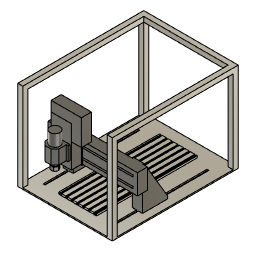
FluidNC Refit Machine Model (Autodesk Fusion 360 design; units mm, degrees)
Autodesk Fusion 360 part; units mm, degrees
sketch "Sketch1" plane through (0, 0, 0) normal (0, 0, 1) x (1, 0, 0) in component "base"
  line L0 (-100, -100) -> (650, -100)
  line L1 (650, -100) -> (650, 900)
  line L2 (650, 900) -> (-100, 900)
  line L3 (-100, 900) -> (-100, -100)
  dimension "d1" = 750
  dimension "d2" = 1000
  dimension "d3" = 100
  dimension "d4" = 100
  constraint horizontal L0
  constraint vertical L1
  constraint horizontal L2
  constraint vertical L3
  measures "d1" distance of L0.start L0.end
  measures "d2" distance of L0.start L2.end
  measures "d3" distance of origin L3
  measures "d4" distance of origin L0
extrude "Extrude1" add sketch "Sketch1" against normal blind 10 makes body 1 in component "base"
ref_plane "WorkPlane1" through (275, 400, -5) normal (-1, 0, 0) x (0, 1, 0)
ref_plane "WorkPlane2" through (275, 400, -5) normal (0, 1, 0) x (1, 0, 0)
sketch "Sketch2" plane through (0, 0, 0) normal (0, 1, 0) x (1, 0, 0) in component "base"
  line L0 (0, 0) -> (125, 0) construction
  line L1 (125, 0) -> (425, 0)
  line L2 (650, 10) -> (-100, 10) construction
  line L3 (275, 0) -> (275, 10) construction
  line L4 (425, 0) -> (425, -15)
  line L5 (425, -15) -> (125, -15) construction
  line L6 (125, -15) -> (125, 0)
  line L7 (275, 0) -> (275, -15) construction
  line L8 (279.15, -15) -> (279.15, -10.6)
  line L9 (279.15, -10.6) -> (282.5, -10.6)
  line L10 (282.5, -10.6) -> (282.5, -4.4)
  line L11 (282.5, -4.4) -> (267.5, -4.4)
  line L12 (267.5, -4.4) -> (267.5, -10.6)
  line L13 (267.5, -10.6) -> (270.85, -10.6)
  line L14 (270.85, -10.6) -> (270.85, -15)
  line L15 (270.85, -10.6) -> (279.15, -10.6) construction
  line L16 (279.15, -15) -> (297.5, -15)
  line L17 (270.85, -15) -> (252.5, -15)
  line L18 (144.15, -15) -> (162.5, -15)
  line L19 (144.15, -15) -> (144.15, -10.6)
  line L20 (144.15, -10.6) -> (147.5, -10.6)
  line L21 (147.5, -4.4) -> (132.5, -4.4)
  line L22 (132.5, -4.4) -> (132.5, -10.6)
  line L23 (132.5, -10.6) -> (135.85, -10.6)
  line L24 (135.85, -10.6) -> (135.85, -15)
  line L25 (135.85, -15) -> (117.5, -15)
  line L26 (147.5, -10.6) -> (147.5, -4.4)
  line L27 (189.15, -15) -> (207.5, -15)
  line L28 (189.15, -15) -> (189.15, -10.6)
  line L29 (189.15, -10.6) -> (192.5, -10.6)
  line L30 (192.5, -4.4) -> (177.5, -4.4)
  line L31 (177.5, -4.4) -> (177.5, -10.6)
  line L32 (177.5, -10.6) -> (180.85, -10.6)
  line L33 (180.85, -10.6) -> (180.85, -15)
  line L34 (180.85, -15) -> (162.5, -15)
  line L35 (192.5, -10.6) -> (192.5, -4.4)
  line L36 (234.15, -15) -> (252.5, -15)
  line L37 (234.15, -15) -> (234.15, -10.6)
  line L38 (234.15, -10.6) -> (237.5, -10.6)
  line L39 (237.5, -4.4) -> (222.5, -4.4)
  line L40 (222.5, -4.4) -> (222.5, -10.6)
  line L41 (222.5, -10.6) -> (225.85, -10.6)
  line L42 (225.85, -10.6) -> (225.85, -15)
  line L43 (225.85, -15) -> (207.5, -15)
  line L44 (237.5, -10.6) -> (237.5, -4.4)
  line L45 (324.15, -15) -> (342.5, -15)
  line L46 (324.15, -15) -> (324.15, -10.6)
  line L47 (324.15, -10.6) -> (327.5, -10.6)
  line L48 (327.5, -4.4) -> (312.5, -4.4)
  line L49 (312.5, -4.4) -> (312.5, -10.6)
  line L50 (312.5, -10.6) -> (315.85, -10.6)
  line L51 (315.85, -10.6) -> (315.85, -15)
  line L52 (315.85, -15) -> (297.5, -15)
  line L53 (327.5, -10.6) -> (327.5, -4.4)
  line L54 (369.15, -15) -> (387.5, -15)
  line L55 (369.15, -15) -> (369.15, -10.6)
  line L56 (369.15, -10.6) -> (372.5, -10.6)
  line L57 (372.5, -4.4) -> (357.5, -4.4)
  line L58 (357.5, -4.4) -> (357.5, -10.6)
  line L59 (357.5, -10.6) -> (360.85, -10.6)
  line L60 (360.85, -10.6) -> (360.85, -15)
  line L61 (360.85, -15) -> (342.5, -15)
  line L62 (372.5, -10.6) -> (372.5, -4.4)
  line L63 (414.15, -15) -> (432.5, -15)
  line L64 (414.15, -15) -> (414.15, -10.6)
  line L65 (414.15, -10.6) -> (417.5, -10.6)
  line L66 (417.5, -4.4) -> (402.5, -4.4)
  line L67 (402.5, -4.4) -> (402.5, -10.6)
  line L68 (402.5, -10.6) -> (405.85, -10.6)
  line L69 (405.85, -10.6) -> (405.85, -15)
  line L70 (405.85, -15) -> (387.5, -15)
  line L71 (417.5, -10.6) -> (417.5, -4.4)
  point P0 (275, -4.4)
  point P1 (275, -10.6)
  dimension "d7" = 300
  dimension "d8" = 15
  dimension "d9" = 8.3
  dimension "d10" = 10.6
  dimension "d11" = 4.4
  dimension "d12" = 15
  dimension "d13" = 45
  dimension "d16" = 45
  dimension "d17" = 0
  constraint coincident L0.start origin
  constraint horizontal L0
  constraint parallel L0 L1
  constraint midpoint L1 L3.start
  constraint midpoint L2 L3.end
  constraint perpendicular L1 L3
  constraint perpendicular L1 L4
  constraint perpendicular L4 L5
  constraint perpendicular L1 L6
  constraint midpoint L5 L7.end
  constraint coincident L5 L8.start
  constraint perpendicular L5 L8
  constraint perpendicular L8 L9
  constraint perpendicular L5 L10
  constraint perpendicular L7 L11
  constraint perpendicular L11 L12
  constraint perpendicular L12 L13
  constraint coincident L5 L14.end
  constraint perpendicular L5 L14
  constraint perpendicular L8 L15
  constraint midpoint L11 P0
  constraint midpoint L15 P1
  constraint coincident L7 P1
  constraint coincident L7 P0
  constraint coincident L5 L16.end
  constraint coincident L5 L17.end
  constraint equal L16 L17
  measures "d7" distance of L0.end L1.end
  measures "d8" distance of L1.end L4.end
  measures "d9" distance of L8 L14
  measures "d10" distance of L5 L11
  measures "d11" distance of L5 L13
  measures "d12" distance of L10 L12
  measures "d13" distance of L16.end L17.end
extrude "Extrude2" add sketch "Sketch2" along normal blind 800 bodies 1 in component "base"
sketch "Sketch3" plane through (0, 0, 0) normal (0, 0, 1) x (-1, 0, 0) in component "base"
  line L0 (-425, -800) -> (-425, 0)
  line L1 (-425, 0) -> (-125, 0)
  line L2 (-125, 0) -> (-125, -800)
  line L3 (-125, -800) -> (-425, -800)
  line L4 (100, -900) -> (100, 100)
  line L5 (100, 100) -> (-650, 100)
  line L6 (-650, 100) -> (-650, -900)
  line L7 (-650, -900) -> (100, -900)
  line L8 (100, -900) -> (60, -900)
  line L9 (60, -900) -> (60, -860)
  line L10 (60, -860) -> (100, -860)
  line L11 (100, -860) -> (100, -900)
  line L12 (-650, -900) -> (-610, -900)
  line L13 (-610, -900) -> (-610, -860)
  line L14 (-610, -860) -> (-650, -860)
  line L15 (-650, -860) -> (-650, -900)
  line L16 (-650, 100) -> (-610, 100)
  line L17 (-610, 100) -> (-610, 60)
  line L18 (-610, 60) -> (-650, 60)
  line L19 (-650, 60) -> (-650, 100)
  line L20 (100, 100) -> (60, 100)
  line L21 (60, 100) -> (60, 60)
  line L22 (60, 60) -> (100, 60)
  line L23 (100, 60) -> (100, 100)
  line L24 (60, -860) -> (-610, -860) construction
  line L25 (-610, -860) -> (-610, 60) construction
  line L26 (-610, 60) -> (60, 60) construction
  line L27 (60, 60) -> (60, -860) construction
  dimension "d21" = 40
  constraint horizontal L8
  constraint vertical L9
  constraint horizontal L10
  constraint vertical L11
  constraint coincident L4.start L7.end
  constraint horizontal L12
  constraint vertical L13
  constraint horizontal L14
  constraint vertical L15
  constraint coincident L6.end L7.start
  constraint horizontal L16
  constraint vertical L17
  constraint horizontal L18
  constraint vertical L19
  constraint coincident L5.end L6.start
  constraint horizontal L20
  constraint vertical L21
  constraint horizontal L22
  constraint vertical L23
  constraint coincident L4.end L5.start
  constraint horizontal L24
  constraint vertical L25
  constraint horizontal L26
  constraint vertical L27
  constraint coincident L13.end L14.start
  constraint equal L8 L11
  constraint equal L12 L15
  constraint equal L20 L23
  constraint coincident L21.end L22.start
  measures "d21" distance of L4.start L10.end
extrude "Extrude3" add sketch "Sketch3" along normal blind 700 contours L4 L7 L8 L9 L10 L11 | L4 L5 L20 L21 L22 L23 | L6 L7 L12 L13 L14 L15 | L5 L6 L16 L17 L18 L19 bodies 1 in component "base"
sketch "Sketch4" plane through (0, 860, 0) normal (0, -1, 0) x (1, 0, 0) in component "base"
  line L0 (-100, 0) -> (-60, 0)
  line L1 (-60, 0) -> (-60, 700)
  line L2 (-60, 700) -> (-100, 700)
  line L3 (-100, 700) -> (-100, 0)
  line L4 (-100, 700) -> (-60, 700)
  line L5 (-60, 700) -> (-60, 660)
  line L6 (-60, 660) -> (-100, 660)
  line L7 (-100, 660) -> (-100, 700)
  line L8 (610, 700) -> (650, 700) construction
  line L9 (610, 700) -> (650, 700)
  line L10 (650, 700) -> (650, 660)
  line L11 (650, 660) -> (610, 660)
  line L12 (610, 660) -> (610, 700)
  constraint horizontal L4
  constraint vertical L5
  constraint horizontal L6
  constraint vertical L7
  constraint coincident L1 L5.end
  constraint coincident L2.end L3.start
  constraint equal L4 L7
  constraint horizontal L9
  constraint vertical L10
  constraint horizontal L11
  constraint vertical L12
  constraint coincident L8.start L9.start
  constraint coincident L5.end L11
  constraint coincident L8.end L10
extrude "Extrude4" add sketch "Sketch4" along normal blind 920 contours L1 L2 L3 L4 L5 L6 L7 | L9 L10 L11 L12 bodies 1 in component "base"
sketch "Sketch5" plane through (610, 0, 0) normal (-1, 0, 0) x (0, -1, 0) in component "base"
  line L0 (-900, 0) -> (-860, 0)
  line L1 (-860, 0) -> (-860, 660)
  line L2 (-860, 660) -> (60, 660)
  line L3 (60, 660) -> (60, 0)
  line L4 (60, 0) -> (100, 0)
  line L5 (100, 0) -> (100, 700)
  line L6 (100, 700) -> (-900, 700)
  line L7 (-900, 700) -> (-900, 0)
  line L8 (-860, 660) -> (-900, 660)
  line L9 (-860, 660) -> (-860, 700)
  line L10 (60, 660) -> (60, 700)
  line L11 (60, 660) -> (100, 660)
  constraint coincident L1.end L2.start
  constraint coincident L7 L8.end
  constraint perpendicular L7 L8
  constraint coincident L6 L9.end
  constraint perpendicular L6 L9
  constraint coincident L2.end L3.start
  constraint coincident L6 L10.end
  constraint perpendicular L6 L10
  constraint coincident L5 L11.end
  constraint perpendicular L5 L11
extrude "Extrude5" add sketch "Sketch5" along normal blind 670 contours L6 L7 L8 L9 bodies 1 in component "base"
sketch "Sketch6" plane through (0, 0, 0) normal (0, 0, 1) x (-1, 0, 0) in component "base"
  line L0 (-610, -860) -> (-610, -900)
  line L1 (-610, -900) -> (60, -900)
  line L2 (60, -900) -> (60, -860)
  line L3 (60, -860) -> (100, -860)
  line L4 (100, -860) -> (100, 60)
  line L5 (100, 60) -> (60, 60)
  line L6 (60, 60) -> (60, 100)
  line L7 (60, 100) -> (-610, 100)
  line L8 (-610, 60) -> (-650, 60)
  line L9 (-650, 60) -> (-650, -860)
  line L10 (-650, -860) -> (-610, -860)
  line L11 (-425, -800) -> (-425, 0)
  line L12 (-425, 0) -> (-125, 0)
  line L13 (-125, 0) -> (-125, -800)
  line L14 (-125, -800) -> (-425, -800)
  line L15 (7.5, -10) -> (-7.5, -10)
  line L16 (-7.5, -10) -> (-7.5, -760)
  line L17 (-7.5, -760) -> (7.5, -760)
  line L18 (7.5, -760) -> (7.5, -10)
  line L19 (-275, 100) -> (-275, -900) construction
  line L20 (-542.5, -10) -> (-542.5, -760)
  line L21 (-542.5, -760) -> (-557.5, -760)
  line L22 (-557.5, -10) -> (-542.5, -10)
  line L23 (-557.5, -760) -> (-557.5, -10)
  line L24 (-610, 100) -> (-610, 60)
  dimension "d28" = 15
  dimension "d29" = 750
  dimension "d30" = 92.5
  dimension "d31" = 110
  constraint horizontal L15
  constraint vertical L16
  constraint horizontal L17
  constraint vertical L18
  constraint midpoint L7 L19.start
  constraint midpoint L1 L19.end
  constraint symmetric L15.start L19 L22.start
  constraint symmetric L15.end L19 L20.start
  constraint symmetric L16.end L19 L20.end
  constraint symmetric L17.end L19 L21.end
  measures "d28" distance of L15.start L15.end
  measures "d29" distance of L15.start L17.end
  measures "d30" distance of L4 L18
  measures "d31" distance of L7 L15
extrude "Extrude6" cut sketch "Sketch6" against normal blind 10 contours L15 L16 L17 L18 | L20 L21 L22 L23 bodies 1 in component "base"
sketch "Sketch7" plane through (0, 0, 0) normal (0, 0, 1) x (-1, 0, 0) in component "base"
  line L0 (-7.5, -10) -> (7.5, -10)
  line L1 (7.5, -10) -> (7.5, -760)
  line L2 (7.5, -760) -> (-7.5, -760)
  line L3 (-7.5, -760) -> (-7.5, -10)
  line L4 (-542.5, -10) -> (-542.5, -760)
  line L5 (-542.5, -760) -> (-557.5, -760)
  line L6 (-557.5, -760) -> (-557.5, -10)
  line L7 (-557.5, -10) -> (-542.5, -10)
  line L8 (-610, -860) -> (-610, -900)
  line L9 (-610, -900) -> (60, -900)
  line L10 (60, -900) -> (60, -860)
  line L11 (60, -860) -> (100, -860)
  line L12 (100, -860) -> (100, 60)
  line L13 (100, 60) -> (60, 60)
  line L14 (60, 60) -> (60, 100)
  line L15 (60, 100) -> (-610, 100)
  line L16 (-610, 60) -> (-650, 60)
  line L17 (-650, 60) -> (-650, -860)
  line L18 (-650, -860) -> (-610, -860)
  line L19 (-425, -800) -> (-425, 0)
  line L20 (-425, 0) -> (-125, 0)
  line L21 (-125, 0) -> (-125, -800)
  line L22 (-125, -800) -> (-425, -800)
  line L23 (80, -860) -> (80, 60) construction
  line L24 (-630, 60) -> (-630, -860) construction
  line L25 (-610, -880) -> (60, -880) construction
  line L26 (-610, -885) -> (60, -885)
  line L27 (60, -885) -> (60, -875)
  line L28 (60, -875) -> (-610, -875)
  line L29 (-610, -875) -> (-610, -885)
  line L30 (-610, -885) -> (60, -875) construction
  line L31 (60, -885) -> (-610, -875) construction
  line L32 (-635, -860) -> (-625, -860)
  line L33 (-625, -860) -> (-625, 60)
  line L34 (-625, 60) -> (-635, 60)
  line L35 (-635, 60) -> (-635, -860)
  line L36 (-635, -860) -> (-625, 60) construction
  line L37 (-625, -860) -> (-635, 60) construction
  line L38 (85, -860) -> (75, -860)
  line L39 (75, -860) -> (75, 60)
  line L40 (75, 60) -> (85, 60)
  line L41 (85, 60) -> (85, -860)
  line L42 (85, -860) -> (75, 60) construction
  line L43 (75, -860) -> (85, 60) construction
  line L44 (-610, 100) -> (-610, 60)
  point P0 (-275, -880)
  point P1 (-630, -400)
  point P2 (80, -400)
  dimension "d34" = 10
  dimension "d35" = 670
  dimension "d36" = 10
  dimension "d37" = 10
  constraint midpoint L11 L23.start
  constraint midpoint L13 L23.end
  constraint midpoint L16 L24.start
  constraint midpoint L18 L24.end
  constraint midpoint L8 L25.start
  constraint midpoint L10 L25.end
  constraint horizontal L26
  constraint perpendicular L26 L27
  constraint parallel L26 L28
  constraint parallel L27 L29
  constraint coincident L30 P0
  constraint coincident L31 P0
  constraint midpoint L25 P0
  constraint horizontal L32
  constraint perpendicular L32 L33
  constraint parallel L32 L34
  constraint parallel L33 L35
  constraint coincident L36 P1
  constraint coincident L37 P1
  constraint coincident L18 L32.start
  constraint midpoint L24 P1
  constraint horizontal L38
  constraint perpendicular L38 L39
  constraint parallel L38 L40
  constraint parallel L39 L41
  constraint coincident L42 P2
  constraint coincident L43 P2
  constraint coincident L11 L38.start
  constraint midpoint L23 P2
  measures "d34" distance of L26.end L27.end L40.end
  measures "d35" distance of L26.start L26.end
  measures "d36" distance of L32.start L32.end
  measures "d37" distance of L38.start L38.end
extrude "Extrude7" add sketch "Sketch7" along normal blind 660 separate body contours L8 L10 L26 L27 L28 L29 | L16 L18 L32 L33 L34 L35 | L11 L13 L38 L39 L40 L41 makes body 2 at (-85, 246.6667, 220) makes body 3 at (163.3333, 875, 220) makes body 4 at (635, 246.6667, 220) in component "base"
sketch "Sketch1 (2)" plane through (0, 0, 0) normal (1, 0, 0) x (0, 1, 0) in component "y_axis_head"
  line L0 (200, 0) -> (200, 340)
  line L1 (200, 340) -> (210, 340)
  line L2 (210, 340) -> (400, 20)
  line L3 (400, 20) -> (400, 0)
  line L4 (400, 0) -> (200, 0)
  dimension "d40" = 20
  dimension "d41" = 10
  dimension "d42" = 200
  dimension "d43" = 340
  dimension "d50" = 200
  constraint vertical L0
  constraint perpendicular L0 L1
  constraint vertical L3
  constraint perpendicular L0 L4
  constraint coincident L0.start L4.end
  constraint coincident origin L4
  measures "d40" distance of L2.end L3.end
  measures "d41" distance of L0.end L1.end
  measures "d42" distance of L3.end L0.start
  measures "d43" distance of L0.start L0.end
  measures "d50" distance of origin L0
extrude "Extrude1'" add sketch "Sketch1 (2)" along normal blind 40 and the other way blind 40 separate body makes body 5 in component "y_axis_head"
mirror "Mirror1" about plane through (275, 400, -5) normal (-1, 0, 0) of bodies 5 makes body 6 in component "y_axis_head"
sketch "Sketch3 (2)" plane through (0, 0, 0) normal (1, 0, 0) x (0, 1, 0) in component "y_axis_head"
  line L0 (200, 340) -> (210, 340)
  line L1 (200, 0) -> (200, 340)
  line L2 (200, 340) -> (120, 340)
  line L3 (120, 340) -> (120, 180)
  line L4 (120, 180) -> (200, 180)
  line L5 (200, 180) -> (200, 340)
  dimension "d51" = 80
  dimension "d52" = 160
  constraint horizontal L2
  constraint vertical L3
  constraint horizontal L4
  constraint vertical L5
  constraint coincident L0.start L1.end
  measures "d51" distance of L0.start L2.end
  measures "d52" distance of L0.start L4.end
extrude "Extrude2'" add sketch "Sketch3 (2)" along normal blind 630 and the other way blind 80 bodies 5 6 in component "y_axis_head"
sketch "Sketch4 (2)" plane through (0, 0, 0) normal (0, 0, -1) x (1, 0, 0) in component "y_axis_head"
  line L0 (-40, -400) -> (40, -400)
  line L1 (40, -400) -> (40, -200)
  line L2 (40, -200) -> (-40, -200)
  line L3 (-40, -200) -> (-40, -400)
  line L4 (0, -200) -> (0, -400) construction
  line L5 (7.5, -200) -> (-7.5, -200)
  line L6 (-7.5, -200) -> (-7.5, -400)
  line L7 (-7.5, -400) -> (7.5, -400)
  line L8 (7.5, -400) -> (7.5, -200)
  line L9 (7.5, -200) -> (-7.5, -400) construction
  line L10 (-7.5, -200) -> (7.5, -400) construction
  point P0 (0, -300)
  dimension "d57" = 15
  constraint midpoint L2 L4.start
  constraint midpoint L0 L4.end
  constraint horizontal L5
  constraint perpendicular L5 L6
  constraint parallel L5 L7
  constraint parallel L6 L8
  constraint coincident L9 P0
  constraint coincident L10 P0
  constraint midpoint L4 P0
  constraint coincident L0 L7.end
  measures "d57" distance of L6.end L7.end
extrude "Extrude3'" add sketch "Sketch4 (2)" along normal blind 40 contours L0 L2 L5 L6 L7 L8 bodies 5 in component "y_axis_head"
mirror "Mirror2" about plane through (275, 400, -5) normal (-1, 0, 0) of "Extrude3'" in component "y_axis_head"
sketch "Sketch5 (2)" plane through (0, 120, 0) normal (0, -1, 0) x (1, 0, 0) in component "y_axis_head"
  line L0 (-80, 180) -> (630, 180)
  line L1 (630, 180) -> (630, 340)
  line L2 (630, 340) -> (-80, 340)
  line L3 (-80, 340) -> (-80, 180)
  line L4 (-80, 340) -> (-80, 260) construction
  line L5 (-80, 260) -> (-80, 180) construction
  line L6 (-80, 220) -> (630, 220) construction
  line L7 (-80, 300) -> (630, 300) construction
  line L8 (275, 180) -> (275, 340) construction
  line L9 (595, 292.5) -> (-45, 292.5)
  line L10 (-45, 292.5) -> (-45, 307.5)
  line L11 (-45, 307.5) -> (595, 307.5)
  line L12 (595, 307.5) -> (595, 292.5)
  line L13 (595, 292.5) -> (-45, 307.5) construction
  line L14 (-45, 292.5) -> (595, 307.5) construction
  line L15 (595, 227.5) -> (-45, 227.5)
  line L16 (-45, 227.5) -> (-45, 212.5)
  line L17 (-45, 212.5) -> (595, 212.5)
  line L18 (595, 212.5) -> (595, 227.5)
  line L19 (595, 227.5) -> (-45, 212.5) construction
  line L20 (-45, 227.5) -> (595, 212.5) construction
  point P0 (275, 300)
  point P1 (275, 220)
  dimension "d62" = 640
  dimension "d63" = 15
  constraint coincident L2.end L3.start
  constraint midpoint L3 L4.end
  constraint coincident L0.start L3.end
  constraint midpoint L5 L6.start
  constraint coincident L1 L6.end
  constraint perpendicular L1 L6
  constraint midpoint L4 L7.start
  constraint coincident L1 L7.end
  constraint perpendicular L1 L7
  constraint midpoint L0 L8.start
  constraint midpoint L2 L8.end
  constraint horizontal L9
  constraint perpendicular L9 L10
  constraint parallel L9 L11
  constraint parallel L10 L12
  constraint coincident L13 P0
  constraint coincident L14 P0
  constraint midpoint L7 P0
  constraint horizontal L15
  constraint perpendicular L15 L16
  constraint parallel L15 L17
  constraint parallel L16 L18
  constraint coincident L19 P1
  constraint coincident L20 P1
  constraint midpoint L6 P1
  constraint equal L9 L15
  constraint equal L10 L16
  measures "d62" distance of L10.end L11.end
  measures "d63" distance of L9.end L10.end
extrude "Extrude4'" cut sketch "Sketch5 (2)" against normal blind 20 contours L9 L10 L11 L12 | L15 L16 L17 L18 bodies 5 in component "y_axis_head"
sketch "Sketch1 (3)" plane through (0, 120, 0) normal (0, -1, 0) x (1, 0, 0) in component "x_axis_head"
  line L0 (-45, 292.5) -> (-45, 307.5)
  line L1 (-45, 307.5) -> (595, 307.5)
  line L2 (595, 307.5) -> (595, 292.5)
  line L3 (595, 292.5) -> (-45, 292.5)
  line L4 (-45, 227.5) -> (595, 227.5)
  line L5 (595, 227.5) -> (595, 212.5)
  line L6 (595, 212.5) -> (-45, 212.5)
  line L7 (-45, 212.5) -> (-45, 227.5)
  line L8 (-80, 180) -> (630, 180)
  line L9 (630, 180) -> (630, 340)
  line L10 (630, 340) -> (-80, 340)
  line L11 (-80, 340) -> (-80, 180)
  line L12 (-80, 260) -> (35, 260) construction
  line L13 (35, 260) -> (35, 340) construction
  line L14 (-50, 175) -> (120, 175)
  line L15 (120, 175) -> (120, 345)
  line L16 (120, 345) -> (-50, 345)
  line L17 (-50, 345) -> (-50, 175)
  line L18 (-50, 175) -> (120, 345) construction
  line L19 (120, 175) -> (-50, 345) construction
  line L20 (-45, 300) -> (35, 300) construction
  line L21 (110, 292.5) -> (-40, 292.5)
  line L22 (-40, 292.5) -> (-40, 307.5)
  line L23 (-40, 307.5) -> (110, 307.5)
  line L24 (110, 307.5) -> (110, 292.5)
  line L25 (110, 292.5) -> (-40, 307.5) construction
  line L26 (-40, 292.5) -> (110, 307.5) construction
  line L27 (110, 212.5) -> (110, 227.5)
  line L28 (110, 227.5) -> (-40, 227.5)
  line L29 (-40, 212.5) -> (110, 212.5)
  line L30 (-40, 227.5) -> (-40, 212.5)
  point P0 (35, 260)
  point P1 (35, 300)
  dimension "d66" = 170
  dimension "d67" = 170
  dimension "d70" = 150
  constraint midpoint L11 L12.start
  constraint perpendicular L11 L12
  constraint coincident L10 L13.end
  constraint perpendicular L10 L13
  constraint horizontal L14
  constraint perpendicular L14 L15
  constraint parallel L14 L16
  constraint parallel L15 L17
  constraint coincident L18 P0
  constraint coincident L19 P0
  constraint coincident P0 L12.end
  constraint midpoint L0 L20.start
  constraint perpendicular L13 L20
  constraint equal L13 L20
  constraint coincident L13 P1
  constraint horizontal L21
  constraint perpendicular L21 L22
  constraint parallel L21 L23
  constraint parallel L22 L24
  constraint coincident L25 P1
  constraint coincident L26 P1
  constraint coincident P1 L20.end
  constraint coincident L3 L21.start
  constraint symmetric L12 L21.start L27.end
  constraint symmetric L12 L21.end L28.end
  constraint symmetric L12 L22.end L29.start
  constraint symmetric L12 L23.end L27.start
  measures "d66" distance of L15.end L16.end
  measures "d67" distance of L14.end L15.end
  measures "d70" distance of L22.end L23.end
extrude "Extrude1''" add sketch "Sketch1 (3)" along normal blind 5 separate body contours L0 L1 L3 L4 L6 L7 L8 L10 L15 L17 L21 L23 L28 L29 | L0 L1 L3 L22 | L1 L3 L21 L22 L23 L24 | L1 L3 L15 L24 | L4 L6 L15 L27 | L10 L15 L16 L17 | L4 L6 L27 L28 L29 L30 | L4 L6 L7 L30 | L8 L14 L15 L17 makes body 7 in component "x_axis_head"
extrude "Extrude2''" add sketch "Sketch1 (3)" against normal blind 10 contours L1 L3 L21 L22 L23 L24 | L4 L6 L27 L28 L29 L30 bodies 7 in component "x_axis_head"
sketch "Sketch2 (2)" plane through (0, 115, 0) normal (0, -1, 0) x (1, 0, 0) in component "x_axis_head"
  line L0 (-50, 345) -> (-50, 175)
  line L1 (120, 175) -> (120, 345)
  line L2 (35, 340) -> (35, 180) construction
  line L3 (35, 260) -> (-50, 260) construction
  line L4 (0, 320) -> (-15, 320)
  line L5 (-15, 320) -> (-15, 200)
  line L6 (-15, 200) -> (0, 200)
  line L7 (0, 200) -> (0, 320)
  line L8 (0, 320) -> (-15, 200) construction
  line L9 (-15, 320) -> (0, 200) construction
  line L10 (85, 320) -> (85, 200)
  line L11 (85, 200) -> (70, 200)
  line L12 (70, 320) -> (85, 320)
  line L13 (70, 200) -> (70, 320)
  line L14 (-50, 175) -> (120, 175)
  line L15 (120, 345) -> (-50, 345)
  point P0 (-7.5, 260)
  dimension "d73" = 15
  dimension "d74" = 120
  constraint midpoint L2 L3.start
  constraint midpoint L0 L3.end
  constraint horizontal L4
  constraint perpendicular L4 L5
  constraint parallel L4 L6
  constraint parallel L5 L7
  constraint coincident L8 P0
  constraint coincident L9 P0
  constraint midpoint L3 P0
  constraint symmetric L2 L4.start L12.start
  constraint symmetric L2 L4.end L10.start
  constraint symmetric L2 L5.end L10.end
  constraint symmetric L2 L6.end L11.end
  measures "d73" distance of L5.end L6.end
  measures "d74" distance of L4.end L5.end
extrude "Extrude3''" add sketch "Sketch2 (2)" along normal blind 10 contours L4 L5 L6 L7 | L10 L11 L12 L13 bodies 7 in component "x_axis_head"
sketch "Sketch3 (3)" plane through (0, 115, 0) normal (0, -1, 0) x (1, 0, 0) in component "z_axis_head"
  line L0 (70, 200) -> (70, 320)
  line L1 (70, 320) -> (85, 320)
  line L2 (85, 320) -> (85, 200)
  line L3 (85, 200) -> (70, 200)
  line L4 (0, 200) -> (-15, 200)
  line L5 (-15, 200) -> (-15, 320)
  line L6 (-15, 320) -> (0, 320)
  line L7 (0, 320) -> (0, 200)
  line L8 (-50, 345) -> (-50, 175)
  line L9 (-50, 175) -> (120, 175)
  line L10 (120, 175) -> (120, 345)
  line L11 (120, 345) -> (-50, 345)
  line L12 (-50, 260) -> (120, 260) construction
  line L13 (115, 420) -> (-45, 420)
  line L14 (-45, 420) -> (-45, 100)
  line L15 (-45, 100) -> (115, 100)
  line L16 (115, 100) -> (115, 420)
  line L17 (115, 420) -> (-45, 100) construction
  line L18 (-45, 420) -> (115, 100) construction
  line L19 (-7.5, 320) -> (-7.5, 200) construction
  line L20 (77.5, 320) -> (77.5, 200) construction
  line L21 (0, 400) -> (-15, 400)
  line L22 (-15, 400) -> (-15, 120)
  line L23 (-15, 120) -> (0, 120)
  line L24 (0, 120) -> (0, 400)
  line L25 (0, 400) -> (-15, 120) construction
  line L26 (-15, 400) -> (0, 120) construction
  line L27 (35, 260) -> (35, 420) construction
  line L28 (70, 120) -> (70, 400)
  line L29 (70, 400) -> (85, 400)
  line L30 (85, 120) -> (70, 120)
  line L31 (85, 400) -> (85, 120)
  point P0 (35, 260)
  point P1 (-7.5, 260)
  dimension "d77" = 320
  dimension "d78" = 160
  dimension "d79" = 15
  dimension "d80" = 280
  constraint midpoint L8 L12.start
  constraint midpoint L10 L12.end
  constraint horizontal L13
  constraint perpendicular L13 L14
  constraint parallel L13 L15
  constraint parallel L14 L16
  constraint coincident L17 P0
  constraint coincident L18 P0
  constraint midpoint L12 P0
  constraint midpoint L6 L19.start
  constraint midpoint L4 L19.end
  constraint midpoint L1 L20.start
  constraint midpoint L3 L20.end
  constraint horizontal L21
  constraint perpendicular L21 L22
  constraint parallel L21 L23
  constraint parallel L22 L24
  constraint coincident L25 P1
  constraint coincident L26 P1
  constraint midpoint L19 P1
  constraint coincident P0 L27.start
  constraint midpoint L13 L27.end
  constraint symmetric L21.start L27 L28.end
  constraint symmetric L21.end L27 L29.end
  constraint symmetric L22.end L27 L30.start
  constraint symmetric L23.end L27 L28.start
  measures "d77" distance of L13.end L14.end
  measures "d78" distance of L13.start L13.end
  measures "d79" distance of L22.end L23.end
  measures "d80" distance of L21.end L22.end
extrude "Extrude1'''" add sketch "Sketch3 (3)" along normal blind 80 separate body contours L0 L7 L9 L11 L24 L28 | L0 L1 L2 L3 L28 L31 | L3 L9 L28 L31 | L1 L11 L28 L31 | L2 L9 L11 L16 L31 | L9 L14 L15 L16 L22 L23 L24 L28 L30 L31 | L9 L28 L30 L31 | L11 L28 L29 L31 | L11 L13 L14 L16 L21 L22 L24 L28 L29 L31 | L9 L22 L23 L24 | L4 L9 L22 L24 | L6 L11 L22 L24 | L11 L21 L22 L24 | L5 L9 L11 L14 L22 | L4 L5 L6 L7 L22 L24 makes body 8 in component "z_axis_head"
extrude "Extrude2'''" cut sketch "Sketch3 (3)" along normal blind 10 contours L0 L1 L2 L3 L28 L31 | L3 L9 L28 L31 | L1 L11 L28 L31 | L9 L28 L30 L31 | L11 L28 L29 L31 | L9 L22 L23 L24 | L4 L9 L22 L24 | L6 L11 L22 L24 | L11 L21 L22 L24 | L4 L5 L6 L7 L22 L24 bodies 8 in component "z_axis_head"
sketch "Sketch1 (4)" plane through (0, 0, 100) normal (0, 0, -1) x (1, 0, 0) in component "z_axis_head"
  line L0 (-45, -115) -> (115, -115)
  line L1 (115, -115) -> (115, -35)
  line L2 (115, -35) -> (-45, -35)
  line L3 (-45, -35) -> (-45, -115)
  line L4 (35, -35) -> (35, 15) construction
  circle A0 centre (35, 15) radius 40
  circle A1 centre (35, 15) radius 60 construction
  line L5 (-20, 38.9792) -> (-20, -20)
  line L6 (-20, -20) -> (-35, -20)
  line L7 (-35, -20) -> (-35, -35)
  line L8 (-35, -35) -> (105, -35)
  line L9 (-20, 38.9792) -> (11.0208, 70)
  line L10 (11.0208, 70) -> (58.9792, 70)
  line L11 (90, 38.9792) -> (58.9792, 70)
  line L12 (90, 38.9792) -> (90, -20)
  line L13 (90, -20) -> (105, -20)
  line L14 (105, -20) -> (105, -35)
  dimension "d85" = 80
  dimension "d86" = 50
  dimension "d87" = 120
  dimension "d88" = 45
  dimension "d89" = 110
  dimension "d90" = 140
  dimension "d91" = 15
  constraint midpoint L2 L4.start
  constraint perpendicular L2 L4
  constraint coincident L4.end A0.centre
  constraint concentric A0 A1
  constraint coincident A1 L5.start
  constraint vertical L5
  constraint perpendicular L5 L6
  constraint coincident L2 L7.end
  constraint perpendicular L2 L7
  constraint coincident L2 L8.end
  constraint midpoint L4.start L8
  constraint coincident A1 L9.end
  constraint coincident A1 L10.end
  constraint perpendicular L5 L10
  constraint symmetric L4 L5.start L11.start
  constraint symmetric L4 L5.end L12.end
  constraint symmetric L4 L6.end L13.end
  constraint symmetric L4 L7.end L8.end
  constraint symmetric L4 L9.end L10.end
  measures "d85" diameter of A0
  measures "d86" distance of L4.start L4.end
  measures "d87" diameter of A1
  measures "d88" angle of L9 L10
  measures "d89" distance of L5 L12
  measures "d90" distance of L7 L14
  measures "d91" distance of L13.end L8.end
extrude "Extrude3'''" add sketch "Sketch1 (4)" against normal blind 110 from surface at -60 separate body contours L2 L5 L6 L7 L8 L9 L10 L11 L12 L13 L14 makes body 9 in component "z_axis_head"
sketch "Sketch2 (3)" plane through (0, 0, 160) normal (0, 0, -1) x (1, 0, 0) in component "z_axis_head"
  circle A0 centre (35, 15) radius 40
  line L0 (90, 38.9792) -> (58.9792, 70)
  line L1 (58.9792, 70) -> (11.0208, 70)
  line L2 (11.0208, 70) -> (-20, 38.9792)
  line L3 (-20, 38.9792) -> (-20, -20)
  line L4 (-20, -20) -> (-35, -20)
  line L5 (-35, -20) -> (-35, -35)
  line L6 (-35, -35) -> (105, -35)
  line L7 (105, -35) -> (105, -20)
  line L8 (105, -20) -> (90, -20)
  line L9 (90, -20) -> (90, 38.9792)
extrude "Extrude4''" add sketch "Sketch2 (3)" along normal blind 10 and the other way blind 204 separate body contours A0 makes body 10 in component "z_axis_head"
sketch "Sketch3 (1)" plane through (0, 0, 150) normal (0, 0, -1) x (1, 0, 0) in component "z_axis_head"
  circle A0 centre (35, 15) radius 40
  circle A1 centre (35, 15) radius 20
  dimension "d99" = 40
  constraint concentric A0 A1
  measures "d99" diameter of A1
extrude "Extrude5'" add sketch "Sketch3 (1)" along normal blind 56 contours A1 bodies 10 in component "z_axis_head"
sketch "Sketch4 (3)" plane through (0, 0, 94) normal (0, 0, -1) x (1, 0, 0) in component "z_axis_head"
  circle A0 centre (35, 15) radius 20
  line L0 (20.5662, 40) -> (6.1325, 15)
  line L1 (6.1325, 15) -> (20.5662, -10)
  line L2 (20.5662, -10) -> (49.4338, -10)
  line L3 (49.4338, -10) -> (63.8675, 15)
  line L4 (63.8675, 15) -> (49.4338, 40)
  line L5 (49.4338, 40) -> (20.5662, 40)
  point P0 (35, 15)
  dimension "d102" = 25
  constraint coincident P0 A0.centre
  constraint horizontal L5
  measures "d102" distance of P0 L5
extrude "Extrude6'" add sketch "Sketch4 (3)" against normal blind 30 bodies 10 in component "z_axis_head"
ref_plane "WorkPlane1" through (63.8675, -15, 94) normal (0, 1, 0) x (-1, 0, 0) in component "z_axis_head"
sketch "Sketch5 (3)" plane through (63.8675, -15, 94) normal (0, 1, 0) x (1, 0, 0) in component "z_axis_head"
  line L0 (-57.735, 0) -> (-57.735, -30)
  line L1 (-57.735, -2.8868) -> (-52.735, 0)
  line L2 (-52.735, 0) -> (-57.735, 0)
  point P0 (-28.8675, 0)
  dimension "d105" = 30
  dimension "d106" = 5
  constraint coincident L0 L1.start
  constraint coincident L0.start L2.end
  constraint perpendicular L0 L2
  measures "d105" angle of L1 L2
  measures "d106" distance of L1.end L0.start
revolve "Revolve1" cut sketch "Sketch5 (3)" angle 360 about axis through (35, -15, 168) along (0, 0, -1) bodies 10 in component "z_axis_head"
sketch "Sketch6 (2)" plane through (0, 0, 420) normal (0, 0, 1) x (-1, 0, 0) in component "z_axis_head"
  line L0 (-115, -115) -> (45, -115)
  line L1 (45, -115) -> (45, -35)
  line L2 (45, -35) -> (-115, -35)
  line L3 (-115, -35) -> (-115, -115)
  line L4 (-115, -115) -> (-195, -115)
  line L5 (-195, -115) -> (-195, -35)
  line L6 (-195, -35) -> (-115, -35)
  line L7 (-115, -35) -> (-115, -115)
  dimension "d108" = 80
  dimension "d109" = 80
  constraint horizontal L4
  constraint vertical L5
  constraint horizontal L6
  constraint vertical L7
  constraint coincident L0.start L3.end
  measures "d108" distance of L0.start L4.end
  measures "d109" distance of L0.start L2.end
extrude "Extrude7'" add sketch "Sketch6 (2)" against normal blind 125 separate body contours L3 L4 L5 L6 L7 makes body 11 in component "z_axis_head"
extrude "Extrude8" add sketch "Sketch6 (2)" along normal blind 80 bodies 11 in component "z_axis_head"
ref_plane "WorkPlane3" through (275, 210, 7.5) normal (0, -1, 0) x (-1, 0, 0)
component "base" placed x (1, 0, 0) y (0, 1, 0) z (0, 0, 1) at (0, 0, 0)
component "y_axis_head" placed x (1, 0, 0) y (0, 1, 0) z (0, 0, 1) at (0, 0, 0)
component "x_axis_head" placed x (1, 0, 0) y (0, 1, 0) z (0, 0, 1) at (75, 0, 0)
component "z_axis_head" placed x (1, 0, 0) y (0, 1, 0) z (0, 0, 1) at (75, 0, 80)
hidden bodies 2 3 4
equation "d10 = 6.2 mm + 4.4 mm"
named bodies: "base", "left window", "rear window", "right window"
